Autodesk Fusion 360 part; units mm, degrees
(part 2 of 2)
sketch "Sketch3" plane through (0, -10, 0) normal (0, -1, 0) x (1, 0, 0)
  line L0 (21.0214, -90) -> (-145.5051, -90)
  line L1 (-145.5051, -90) -> (-145.5051, -110)
  line L2 (-145.5051, -110) -> (21.0214, -110)
  line L3 (21.0214, -110) -> (42.6768, -147.5083)
  line L4 (42.6768, -160) -> (62.6768, -160)
  line L5 (62.6768, -142.1493) -> (38.3419, -100)
  line L6 (38.3419, -100) -> (63.4081, -56.584)
  line L7 (63.4081, -56.584) -> (53.416, -19.2927)
  line L8 (53.416, -19.2927) -> (5, 8.6603)
  line L9 (5, 8.6603) -> (-5, -8.6603)
  line L10 (-5, -8.6603) -> (36.2416, -32.4711)
  line L11 (36.2416, -32.4711) -> (41.9455, -53.7584)
  line L12 (41.9455, -53.7584) -> (21.0214, -90)
  line L13 (49.8889, -160) -> (82.45, -160)
  line L14 (82.45, -160) -> (110.5593, -200.6722)
  line L15 (110.5593, -200.6722) -> (43.8339, -200.6722)
  line L16 (43.8339, -200.6722) -> (49.8889, -160)
  line L17 (67.2094, -160) -> (67.2094, -150)
  line L18 (42.6768, -147.5083) -> (42.6768, -160)
  line L19 (62.6768, -160) -> (62.6768, -142.1493)
  dimension "d24" = 50
  dimension "d28" = 10
  constraint coincident L3 L13.start
  constraint horizontal L13
  constraint parallel L13 L15
  constraint coincident L13 L17.start
  constraint coincident L5 L17.end
  constraint perpendicular L13 L17
  measures "d24" vertical distance of L2.end L13.start
  measures "d28" distance of L17.start L17.end
sketch "Sketch4" plane through (0, 0, -90) normal (0, 0, 1) x (-1, 0, 0)
  line L0 (-21.0214, 10) -> (-21.0214, -10)
  line L1 (-21.0214, -10) -> (145.5051, -10)
  line L2 (145.5051, -10) -> (145.5051, 10)
  line L3 (145.5051, 10) -> (-21.0214, 10)
  line L4 (145.5051, 0) -> (43.2223, 0) construction
  circle A0 centre (138.0051, 0) radius 2
  circle A1 centre (123.0051, 0) radius 2
  line L5 (141.7051, -2.1362) -> (141.7051, 2.1362)
  line L6 (141.7051, 2.1362) -> (138.0051, 4.2724)
  line L7 (138.0051, 4.2724) -> (134.3051, 2.1362)
  line L8 (134.3051, 2.1362) -> (134.3051, -2.1362)
  line L9 (134.3051, -2.1362) -> (138.0051, -4.2724)
  line L10 (138.0051, -4.2724) -> (141.7051, -2.1362)
  line L11 (126.7051, -2.1362) -> (126.7051, 2.1362)
  line L12 (126.7051, 2.1362) -> (123.0051, 4.2724)
  line L13 (123.0051, 4.2724) -> (119.3051, 2.1362)
  line L14 (119.3051, 2.1362) -> (119.3051, -2.1362)
  line L15 (119.3051, -2.1362) -> (123.0051, -4.2724)
  line L16 (123.0051, -4.2724) -> (126.7051, -2.1362)
  point P0 (138.0051, 0)
  point P1 (123.0051, 0)
  dimension "d31" = 4
  dimension "d32" = 7.5
  dimension "d33" = 15
  dimension "d34" = 7.4
  constraint midpoint L2 L4.start
  constraint perpendicular L2 L4
  constraint coincident L4 P0
  constraint coincident L4 P1
  constraint equal A0 A1
  constraint coincident P0 A0.centre
  constraint coincident P1 A1.centre
  constraint vertical L5
  constraint vertical L11
  constraint horizontal L9.end L15.end
  measures "d31" diameter of A0
  measures "d32" distance of L4.start P0
  measures "d33" distance of P0 P1
  measures "d34" distance of L5 L8
extrude "Extrude4" cut sketch "Sketch4" against normal blind 50 contours A0 | A1
extrude "Extrude5" cut sketch "Sketch4" against normal blind 5 contours L5 L6 L7 L8 L9 L10 | L11 L12 L13 L14 L15 L16
equation "d19 = 7 mm + 2 * gap"
equation "gap = 0.2 mm"
equation "d34 = 7 mm + 2 * gap"

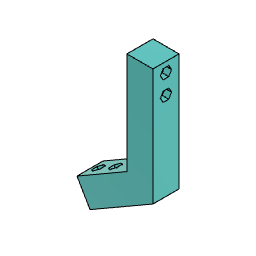
design "upper_middle_frame"
Autodesk Fusion 360 part; units mm, degrees
sketch "Sketch1" plane through (0, 0, 0) normal (0, 1, 0) x (1, 0, 0)
  line L0 (0, 0) -> (26.1117, 0) construction
  line L1 (0, 0) -> (43.3013, -25)
  line L2 (43.3013, -25) -> (43.3013, -109)
  dimension "d1" = 50
  dimension "d2" = 30
  dimension "d3" = 84
  constraint coincident L0.start L1.start
  constraint horizontal L0
  constraint perpendicular L0 L2
  measures "d1" distance of L0.start L1.end
  measures "d2" angle of L0 L1
  measures "d3" distance of L1.end L2.end
pipe "Pipe1" add square section size 20 path "Sketch1" along L1 L2
sketch "Sketch2" plane through (-5, 0, 8.6603) normal (-0.5, 0, 0.866025) x (0, -1, 0)
  line L0 (-10, 0) -> (10, 0)
  line L1 (10, 0) -> (10, 44.2265)
  line L2 (10, 44.2265) -> (-10, 44.2265)
  line L3 (-10, 44.2265) -> (-10, 0)
  line L4 (0, 0) -> (0, 44.2265) construction
  circle A0 centre (0, 7.5) radius 2
  circle A1 centre (0, 22.5) radius 2
  line L5 (2.1362, 3.8) -> (4.2724, 7.5)
  line L6 (4.2724, 7.5) -> (2.1362, 11.2)
  line L7 (2.1362, 11.2) -> (-2.1362, 11.2)
  line L8 (-2.1362, 11.2) -> (-4.2724, 7.5)
  line L9 (-4.2724, 7.5) -> (-2.1362, 3.8)
  line L10 (-2.1362, 3.8) -> (2.1362, 3.8)
  line L11 (2.1362, 18.8) -> (4.2724, 22.5)
  line L12 (4.2724, 22.5) -> (2.1362, 26.2)
  line L13 (2.1362, 26.2) -> (-2.1362, 26.2)
  line L14 (-2.1362, 26.2) -> (-4.2724, 22.5)
  line L15 (-4.2724, 22.5) -> (-2.1362, 18.8)
  line L16 (-2.1362, 18.8) -> (2.1362, 18.8)
  point P0 (0, 7.5)
  point P1 (0, 22.5)
  dimension "d8" = 4
  dimension "d9" = 7.5
  dimension "d10" = 15
  dimension "d11" = 7.4
  constraint coincident L4.start origin
  constraint midpoint L2 L4.end
  constraint coincident L4 P0
  constraint coincident L4 P1
  constraint equal A0 A1
  constraint coincident P0 A0.centre
  constraint coincident P1 A1.centre
  constraint vertical L5.end L11.end
  constraint horizontal L10
  constraint horizontal L16
  measures "d8" diameter of A1
  measures "d9" distance of L4.start A0.centre
  measures "d10" distance of P0 P1
  measures "d11" distance of L7 L10
extrude "Extrude1" cut sketch "Sketch2" against normal blind 40 contours A0 | A1
extrude "Extrude2" cut sketch "Sketch2" against normal blind 5 contours L5 L6 L7 L8 L9 L10 | L11 L12 L13 L14 L15 L16
sketch "Sketch3" plane through (53.3013, 0, 0) normal (1, 0, 0) x (0, 1, 0)
  line L0 (-10, 19.2265) -> (10, 19.2265)
  line L1 (10, 19.2265) -> (10, 109)
  line L2 (10, 109) -> (-10, 109)
  line L3 (-10, 109) -> (-10, 19.2265)
  line L4 (0, 109) -> (0, 74.4412) construction
  circle A0 centre (0, 101.5) radius 2
  circle A1 centre (0, 86.5) radius 2
  line L5 (-2.1362, 105.2) -> (-4.2724, 101.5)
  line L6 (-4.2724, 101.5) -> (-2.1362, 97.8)
  line L7 (-2.1362, 97.8) -> (2.1362, 97.8)
  line L8 (2.1362, 97.8) -> (4.2724, 101.5)
  line L9 (4.2724, 101.5) -> (2.1362, 105.2)
  line L10 (2.1362, 105.2) -> (-2.1362, 105.2)
  line L11 (-2.1362, 90.2) -> (-4.2724, 86.5)
  line L12 (-4.2724, 86.5) -> (-2.1362, 82.8)
  line L13 (-2.1362, 82.8) -> (2.1362, 82.8)
  line L14 (2.1362, 82.8) -> (4.2724, 86.5)
  line L15 (4.2724, 86.5) -> (2.1362, 90.2)
  line L16 (2.1362, 90.2) -> (-2.1362, 90.2)
  point P0 (0, 101.5)
  point P1 (0, 86.5)
  dimension "d17" = 4
  dimension "d18" = 7.5
  dimension "d19" = 15
  dimension "d20" = 7.4
  constraint midpoint L2 L4.start
  constraint perpendicular L2 L4
  constraint coincident L4 P0
  constraint coincident L4 P1
  constraint equal A0 A1
  constraint coincident P0 A0.centre
  constraint coincident P1 A1.centre
  constraint equal L10 L16
  constraint horizontal L10
  constraint horizontal L16
  measures "d17" diameter of A0
  measures "d18" distance of L4.start P0
  measures "d19" distance of P0 P1
  measures "d20" distance of L7 L10
extrude "Extrude3" cut sketch "Sketch3" against normal blind 55 contours A0 | A1
extrude "Extrude4" cut sketch "Sketch3" against normal blind 5 contours L5 L6 L7 L8 L9 L10 | L11 L12 L13 L14 L15 L16
equation "d11 = 7 mm + 2 * gap"
equation "gap = 0.2 mm"
equation "d20 = 7 mm + 2 * gap"

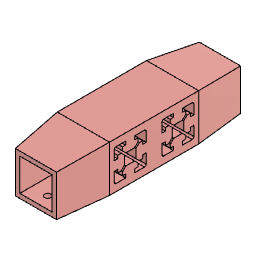
design "upper_double_connector"
Autodesk Fusion 360 part; units mm, degrees
sketch "Sketch1" plane through (0, 0, 0) normal (1, 0, 0) x (0, 1, 0)
  line L0 (7.9, 2.9) -> (7.9, 4.9)
  line L1 (-2.7515, -3.6) -> (-4.9, -5.7485)
  line L2 (2.9, -7.9) -> (4.9, -7.9)
  line L3 (-2.9, -7.9) -> (-2.9, -10.1)
  arc A0 (-10.1, -9) -> (-9, -10.1) centre (-9, -9) ccw
  line L4 (5.7485, 4.9) -> (3.6, 2.7515)
  line L5 (-7.9, 2.9) -> (-10.1, 2.9)
  line L6 (-4.9, -7.9) -> (-2.9, -7.9)
  line L7 (4.9, 5.7485) -> (4.9, 7.9)
  line L8 (10.1, 2.9) -> (7.9, 2.9)
  line L9 (9, -10.1) -> (2.9, -10.1)
  arc A1 (9, -10.1) -> (10.1, -9) centre (9, -9) ccw
  line L10 (4.9, -5.7485) -> (2.7515, -3.6)
  line L11 (5.7485, -4.9) -> (7.9, -4.9)
  line L12 (-10.1, 2.9) -> (-10.1, 9)
  line L13 (7.9, -2.9) -> (10.1, -2.9)
  line L14 (-3.6, 2.7515) -> (-5.7485, 4.9)
  line L15 (10.1, -2.9) -> (10.1, -9)
  line L16 (-2.9, 10.1) -> (-2.9, 7.9)
  line L17 (7.9, -4.9) -> (7.9, -2.9)
  line L18 (-3.6, -2.7515) -> (-3.6, 2.7515)
  line L19 (3.6, 2.7515) -> (3.6, -2.7515)
  line L20 (2.7515, -3.6) -> (-2.7515, -3.6)
  line L21 (-10.1, -9) -> (-10.1, -2.9)
  line L22 (10.1, 9) -> (10.1, 2.9)
  line L23 (2.9, 7.9) -> (2.9, 10.1)
  line L24 (7.9, 4.9) -> (5.7485, 4.9)
  line L25 (-2.9, -10.1) -> (-9, -10.1)
  line L26 (-2.7515, 3.6) -> (2.7515, 3.6)
  arc A2 (-9, 10.1) -> (-10.1, 9) centre (-9, 9) ccw
  line L27 (4.9, 7.9) -> (2.9, 7.9)
  line L28 (-7.9, -4.9) -> (-5.7485, -4.9)
  line L29 (2.9, 10.1) -> (9, 10.1)
  arc A3 (10.1, 9) -> (9, 10.1) centre (9, 9) ccw
  line L30 (-4.9, -5.7485) -> (-4.9, -7.9)
  line L31 (-7.9, -2.9) -> (-7.9, -4.9)
  line L32 (-4.9, 7.9) -> (-4.9, 5.7485)
  line L33 (2.7515, 3.6) -> (4.9, 5.7485)
  line L34 (-4.9, 5.7485) -> (-2.7515, 3.6)
  line L35 (-10.1, -2.9) -> (-7.9, -2.9)
  line L36 (3.6, -2.7515) -> (5.7485, -4.9)
  line L37 (4.9, -7.9) -> (4.9, -5.7485)
  line L38 (2.9, -10.1) -> (2.9, -7.9)
  line L39 (-5.7485, -4.9) -> (-3.6, -2.7515)
  line L40 (-7.9, 4.9) -> (-7.9, 2.9)
  line L41 (-2.9, 7.9) -> (-4.9, 7.9)
  line L42 (-9, 10.1) -> (-2.9, 10.1)
  line L43 (-5.7485, 4.9) -> (-7.9, 4.9)
  line L44 (-15.1, 14.6) -> (13.1, 14.6)
  line L45 (13.1, 14.6) -> (13.1, -14.6)
  line L46 (13.1, -14.6) -> (-15.1, -14.6)
  line L47 (-15.1, -14.6) -> (-15.1, 14.6)
  dimension "d25" = 4.5
  dimension "d26" = 4.5
  dimension "d27" = 3
  dimension "d28" = 5
  constraint horizontal L44
  constraint vertical L45
  constraint horizontal L46
  constraint vertical L47
  measures "d25" distance of L42 L44
  measures "d26" distance of L9 L46
  measures "d27" distance of L22 L45
  measures "d28" distance of L12 L47
extrude "Extrude1" add sketch "Sketch1" along normal blind 3 contours L0 L1 L2 L3 A0 L4 L5 L6 L7 L8 L9 A1 L10 L11 L12 L13 L14 L15 L16 L17 L18 L19 L20 L21 L22 L23 L24 L25 L26 A2 L27 L28 L29 A3 L30 L31 L32 L33 L34 L35 L36 L37 L38 L39 L40 L41 L42 L43 | L44 L45 L46 L47
extrude "Extrude2" add sketch "Sketch1" along normal blind 30 from surface at 3
ref_plane "WorkPlane1" through (16.5, 43.1, 0) normal (0, 1, 0) x (0, 0, 1)
sketch "Sketch2" plane through (0, 43.1, 0) normal (0, 1, 0) x (1, 0, 0)
  line L0 (29.5, 14.6) -> (3.5, 14.6)
  line L1 (3.5, 14.6) -> (3.5, -11.4)
  line L2 (3.5, -11.4) -> (29.5, -11.4)
  line L3 (29.5, -11.4) -> (29.5, 14.6)
  line L4 (26.7, 11.8) -> (6.3, 11.8)
  line L5 (6.3, 11.8) -> (6.3, -8.6)
  line L6 (6.3, -8.6) -> (26.7, -8.6)
  line L7 (26.7, -8.6) -> (26.7, 11.8)
  line L8 (16.5, -14.6) -> (16.5, 14.6) construction
  line L9 (0, -14.6) -> (33, -14.6)
  line L10 (0, 14.6) -> (33, 14.6)
  line L11 (0, -14.6) -> (0, 14.6)
  line L12 (33, 14.6) -> (33, -14.6)
  dimension "d15" = 20.4
  dimension "d16" = 20.4
  dimension "d17" = 2.8
  dimension "d18" = 2.8
  dimension "d23" = 2.8
  dimension "d29" = 2.8
  constraint horizontal L0
  constraint vertical L1
  constraint horizontal L2
  constraint vertical L3
  constraint horizontal L4
  constraint vertical L5
  constraint horizontal L6
  constraint vertical L7
  constraint symmetric L1 L3 L8
  constraint midpoint L8.start L9
  constraint midpoint L8.end L10
  constraint collinear L0 L10
  measures "d15" distance of L4.end L5.end
  measures "d16" distance of L5.end L6.end
  measures "d17" distance of L3 L7
  measures "d18" distance of L1 L5
  measures "d23" distance of L2 L6
  measures "d29" distance of L0 L4
loft "Loft1" add profiles "Sketch2" section 1 face at (11, 13.1, 4.8667) section 2 contours L0 L1 L2 L3 L10 | L4 L5 L6 L7
extrude "Extrude3" cut sketch "Sketch2" against normal blind 30 contours L4 L5 L6 L7
sketch "Sketch3" plane through (0, 0, -11.8) normal (0, 0, 1) x (-1, 0, 0)
  line L0 (-26.7, -43.1) -> (-6.3, -43.1)
  line L1 (-6.3, -43.1) -> (-6.3, -13.1)
  line L2 (-6.3, -13.1) -> (-26.7, -13.1)
  line L3 (-26.7, -13.1) -> (-26.7, -43.1)
  line L4 (-16.5, -43.1) -> (-16.5, -13.1) construction
  circle A0 centre (-16.5, -35.6) radius 2
  circle A1 centre (-16.5, -20.6) radius 2
  dimension "d30" = 7.5
  dimension "d31" = 15
  dimension "d32" = 4
  constraint midpoint L0 L4.start
  constraint midpoint L2 L4.end
  constraint coincident L4 A0.centre
  constraint coincident L4 A1.centre
  constraint equal A0 A1
  measures "d30" distance of L4.start A0.centre
  measures "d31" distance of A0.centre A1.centre
  measures "d32" diameter of A1
extrude "Extrude4" cut sketch "Sketch3" against normal blind 5 contours A0 | A1
mirror "Mirror1" about plane through (0, -15.1, -14.6) normal (0, -1, 0) of bodies 1 merged
equation "gap = 0.2 mm"
equation "d15 = 20 mm + 2 * gap"
equation "d16 = 20 mm + 2 * gap"
equation "d17 = 3 mm - gap"
equation "d18 = 3 mm - gap"
equation "d23 = 3 mm - gap"
equation "d29 = 3 mm - gap"
